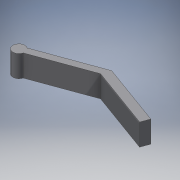
# Autodesk Inventor part: arm1
Saved by Autodesk Inventor 2020 (Build 240168000, 168)
## iProperties
Created: 2020-02-04
Part Number: arm1
Material: Generic
Document SubType Name: Modeling
Designer: Wes
Density: 1 g/cm^3
Appearance: Default
Author: Wes
Autodesk Inventor part; units mm, degrees
ref_plane "YZ Plane" through (0, 0, 0) normal (1, 0, 0) x (0, 1, 0)
ref_plane "XZ Plane" through (0, 0, 0) normal (0, 1, 0) x (-1, 0, 0)
ref_plane "XY Plane" through (0, 0, 0) normal (0, 0, 1) x (1, 0, 0)
sketch "Sketch1 - gripper" plane through (0, 0, 0) normal (0, 0, 1) x (1, 0, 0)
  line L0 (0, 0) -> (-10.2606, -28.1908)
  line L1 (0, 0) -> (30, 0) construction
  line L2 (-10.2606, -28.1908) -> (0, -56.3816)
  line L3 (0, 0) -> (-3.7588, 1.3681)
  line L4 (-3.7588, 1.3681) -> (-14.0194, -26.8227)
  line L5 (-14.0194, -26.8227) -> (-2.8794, -57.4296)
  line L6 (-2.8794, -57.4296) -> (0, -56.3816)
  circle A0 centre (-1.4397, -56.9056) radius 2.75
  point P0 (-3.6605, -55.2836)
  point P1 (-0.7811, -54.2356)
  dimension "d4" = 30
  dimension "d5" = 110
  dimension "d6" = 30
  dimension "d7" = 4
  dimension "d9" = 5.5
  constraints: 14 end point, 2 perpendicular, 1 centre point, 1 equal length, 1 horizontal, 1 midpoint
  measures "d4" distance of L0.start L0.end
  measures "d5" angle of L0 L1
  measures "d6" distance of L0.end L2.end
  measures "d7" distance of L0.start L3.end
  measures "d9" diameter of A0
extrude "Extrusion1" add sketch "Sketch1 - gripper" along normal blind 10
body "Solid2"
